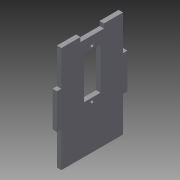
# Autodesk Inventor part: Side
Saved by Autodesk Inventor 2013 (Build 170138000, 138)
## iProperties
Created: 2013-04-20
Part Number: Side
Material: Generic
Document SubType Name: Modeling
Designer: fuji
Density: 1 g/cm^3
Author: fuji
Autodesk Inventor part; units mm, degrees
ref_plane "YZ Plane" through (0, 0, 0) normal (1, 0, 0) x (0, 1, 0)
ref_plane "XZ Plane" through (0, 0, 0) normal (0, 1, 0) x (-1, 0, 0)
ref_plane "XY Plane" through (0, 0, 0) normal (0, 0, 1) x (1, 0, 0)
sketch "Sketch1" plane through (0, 0, 0) normal (1, 0, 0) x (0, 1, 0)
  line L0 (0, 0) -> (76.2, 0)
  line L1 (76.2, 0) -> (76.2, -44.45)
  line L2 (76.2, -44.45) -> (0, -44.45)
  line L3 (0, -44.45) -> (0, 0)
  dimension "d0" = 76.2
  dimension "d1" = 44.45
  constraints: 8 end point, 2 parallel, 1 horizontal, 1 perpendicular
  measures "d0" distance of L1.end L2.end
  measures "d1" distance of L0.end L1.end
extrude "Extrusion1" add sketch "Sketch1" along normal blind 3.175
sketch "Sketch2" plane through (3.175, 0, 0) normal (1, 0, 0) x (0, 0, -1)
  line L0 (44.45, 76.2) -> (0, 76.2) projected
  line L1 (13.7583, 76.2) -> (30.6917, 76.2)
  line L2 (30.6917, 76.2) -> (30.6917, 73.025)
  line L3 (30.6917, 73.025) -> (13.7583, 73.025)
  line L4 (13.7583, 73.025) -> (13.7583, 76.2)
  line L5 (0, 76.2) -> (0, 0) projected
  dimension "d4" = 16.9333
  dimension "d5" = 3.175
  dimension "d8" = 13.7583
  constraints: 8 end point, 2 parallel, 1 horizontal, 1 perpendicular, 1 point on line
  measures "d4" distance of L2.end L3.end
  measures "d5" distance of L1.end L2.end
  measures "d8" distance between parallel lines of L5 L4
extrude "Extrusion2" cut sketch "Sketch2" against normal blind 3.175
sketch "Sketch3" plane through (3.175, 0, 0) normal (1, 0, 0) x (0, 0, -1)
  line L0 (0, 76.2) -> (0, 0) projected
  line L1 (0, 0) -> (44.45, 0) projected
  line L2 (44.45, 0) -> (44.45, 76.2) projected
  line L3 (44.45, 50.8) -> (47.625, 50.8)
  line L4 (47.625, 50.8) -> (47.625, 25.4)
  line L5 (47.625, 25.4) -> (44.45, 25.4)
  line L6 (44.45, 25.4) -> (44.45, 50.8)
  line L7 (0, 50.8) -> (-3.175, 50.8)
  line L8 (-3.175, 50.8) -> (-3.175, 25.4)
  line L9 (-3.175, 25.4) -> (0, 25.4)
  line L10 (0, 25.4) -> (0, 50.8)
  dimension "d9" = 3.175
  dimension "d10" = 25.4
  dimension "d11" = 25.4
  dimension "d12" = 3.175
  dimension "d13" = 25.4
  constraints: 16 end point, 4 parallel, 2 horizontal, 2 perpendicular, 2 point on line, 1 collinear
  measures "d9" distance of L4.end L5.end
  measures "d10" distance of L3.end L4.end
  measures "d11" distance between parallel lines of L1 L5
  measures "d12" distance of L9.end L8.end
  measures "d13" distance of L8.end L7.end
extrude "Extrusion3" add sketch "Sketch3" against normal blind 3.175
sketch "Sketch4" plane through (3.175, 0, 0) normal (1, 0, 0) x (0, 0, -1)
  line L0 (-3.175, 50.8) -> (-3.175, 25.4) projected
  line L1 (44.45, 76.2) -> (30.6917, 76.2) projected
  line L2 (16.225, 64.2) -> (28.225, 64.2)
  line L3 (28.225, 64.2) -> (28.225, 34.2)
  line L4 (28.225, 34.2) -> (16.225, 34.2)
  line L5 (16.225, 34.2) -> (16.225, 64.2)
  circle A0 centre (22.225, 66.7) radius 1.0541
  circle A1 centre (22.225, 31.7) radius 1.0541
  dimension "d16" = 12
  dimension "d17" = 30
  dimension "d19" = 19.4
  dimension "d20" = 12
  dimension "d21" = 2.1082
  dimension "d22" = 6
  dimension "d23" = 2.5
  dimension "d24" = 2.1082
  dimension "d25" = 6
  dimension "d26" = 2.5
  constraints: 8 end point, 2 centre point, 2 parallel, 1 horizontal, 1 perpendicular
  measures "d16" distance of L3.end L4.end
  measures "d17" distance of L2.end L3.end
  measures "d19" distance between parallel lines of L5 L0
  measures "d20" distance between parallel lines of L1 L2
  measures "d21" diameter of A0
  measures "d22" distance from line of A0.centre L5
  measures "d23" distance from line of L2 A0.centre
  measures "d24" diameter of A1
  measures "d25" distance from line of L5 A1.centre
  measures "d26" distance from line of A1.centre L4
extrude "Extrusion4" cut sketch "Sketch4" against normal blind 3.175
equation "\"d0\" = height"
equation "\"d1\" = depth - 2 * thick"
equation "\"d2\" = thick"
equation "\"d4\" = 0.333333 * depth"
equation "\"d5\" = thick"
equation "\"d8\" = 0.333333 * depth - thick"
equation "\"d6\" = thick"
equation "\"d9\" = thick"
equation "\"d10\" = 0.333333 * height"
equation "\"d11\" = 0.333333 * height"
equation "\"d12\" = thick"
equation "\"d13\" = 0.333333 * height"
equation "\"d14\" = thick"
equation "\"d16\" = servoWidth"
equation "\"d17\" = servoLength"
equation "\"d19\" = -0.5 * servoWidth + 0.5 * depth"
equation "\"d20\" = servoOffset"
equation "\"d21\" = servoHole"
equation "\"d22\" = 0.5 * servoWidth"
equation "\"d23\" = -0.5 * servoLength + 0.5 * servoDist"
equation "\"d24\" = servoHole"
equation "\"d25\" = 0.5 * servoWidth"
equation "\"d26\" = -0.5 * servoLength + 0.5 * servoDist"
equation "\"d27\" = thick"
equation "\"height\" = 76.2"
equation "\"thick\" = 3.175"
equation "\"depth\" = 50.8"
equation "\"servoLength\" = 30"
equation "\"servoWidth\" = 12"
equation "\"servoOffset\" = 12"
equation "\"servoDist\" = 35"
equation "\"servoHole\" = 2.1082"
body "Solid1"
